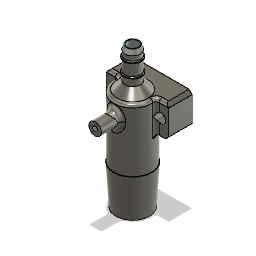
Pneumatic Connectors V2 - Respiratory Pressure V2 (Autodesk Fusion 360 design; units mm, degrees)
Autodesk Fusion 360 part; units mm, degrees
sketch "Sketch1" plane through (0, 0, 0) normal (0, 1, 0) x (1, 0, 0)
  circle A0 centre (0, 0) radius 5
  dimension "d1" = 10
  constraint coincident A0.centre origin
  measures "d1" diameter of A0
  measures "d21" distance of A0.centre
  measures "d24" diameter of A0.centre
  measures "d28" diameter of A0.centre
ref_plane "WorkPlane1" through (0, 15, 0) normal (0, 1, 0) x (1, 0, 0)
sketch "Sketch2" plane through (0, 15, 0) normal (0, 1, 0) x (1, 0, 0)
  circle A0 centre (0, 0) radius 5
  dimension "d3" = 10
  constraint coincident A0.centre origin
  measures "d3" diameter of A0
loft "Loft1" add profiles "Sketch1", "Sketch2" section 1 section 2
sketch "Sketch3" plane through (0, 15, 0) normal (0, 1, 0) x (-1, 0, 0)
  circle A0 centre (0, 0) radius 5
  circle A1 centre (0, 0) radius 3.5
  dimension "d4" = 7
  constraint coincident A0.centre A1.centre
  measures "d4" diameter of A1
sketch "Sketch4" plane through (0, 0, 0) normal (0, -1, 0) x (1, 0, 0)
  circle A0 centre (0, 0) radius 5
  circle A1 centre (0, 0) radius 3.5
  dimension "d5" = 7
  constraint concentric A0 A1
  measures "d5" diameter of A1
loft "Loft2" cut profiles "Sketch3", "Sketch4" section 1 contours A1 section 2 contours A1
sketch "Sketch14" plane through (0, 0, 0) normal (0, -1, 0) x (1, 0, 0)
  circle A0 centre (0, 0) radius 3.5
  circle A1 centre (0, 0) radius 5
  circle A2 centre (0, 0) radius 5
  constraint concentric A0 A2
  constraint equal A1 A2
extrude "Extrude2" add sketch "Sketch14" along normal blind 50
ref_plane "WorkPlane3" through (0, -75, 0) normal (0, -1, 0) x (1, 0, 0)
sketch "Sketch6" plane through (0, -75, 0) normal (0, -1, 0) x (1, 0, 0)
  circle A0 centre (0, 0) radius 10.75
  dimension "d42" = 21.5
  constraint coincident A0.centre origin
  measures "d42" diameter of A0
sketch "Sketch7" plane through (0, -50, 0) normal (0, -1, 0) x (1, 0, 0)
  circle A0 centre (0, 0) radius 3.5
  circle A1 centre (0, 0) radius 5
  circle A2 centre (0, 0) radius 12.25
  dimension "d43" = 24.5
  constraint concentric A0 A2
  measures "d43" diameter of A2
ref_plane "WorkPlane6" through (0, -50, 0) normal (0, -1, 0) x (1, 0, 0)
loft "Loft3" add profiles "Sketch7", "Sketch6" section 1 contours A1 | A2 section 2
sketch "Sketch8" plane through (0, -50, 0) normal (0, -1, 0) x (1, 0, 0)
  circle A0 centre (0, 0) radius 4.5
  dimension "d18" = 9
  constraint coincident A0.centre origin
  measures "d18" diameter of A0
sketch "Sketch15" plane through (0, -75, 0) normal (0, -1, 0) x (1, 0, 0)
  circle A0 centre (0, 0) radius 5.75
  circle A1 centre (0, 0) radius 11.75
  circle A2 centre (0, 0) radius 11.5
  circle A3 centre (0, 0) radius 7
  circle A4 centre (0, 0) radius 10.75
  dimension "d37" = 11.5
  measures "d37" diameter of A0
loft "Loft4" cut profiles "Sketch8", "Sketch15" section 1 section 2 contours A0
ref_plane "WorkPlane8" through (0, -10, 0) normal (0, -1, 0) x (1, 0, 0)
sketch "Sketch10" plane through (0, -10, 0) normal (0, -1, 0) x (1, 0, 0)
  line L0 (0, 0) -> (0, -30.326) construction
  line L1 (20, -3) -> (-20, -3)
  line L2 (-20, -3) -> (-20, -18)
  line L3 (-20, -18) -> (20, -18)
  line L4 (20, -18) -> (20, -3)
  line L5 (20, -3) -> (-20, -18) construction
  line L6 (-20, -3) -> (20, -18) construction
  circle A0 centre (0, 0) radius 5
  circle A1 centre (0, 0) radius 5
  point P0 (0, -10.5)
  dimension "d20" = 15
  dimension "d21" = 40
  constraint coincident L0.start A0.centre
  constraint vertical L0
  constraint horizontal L1
  constraint perpendicular L1 L2
  constraint parallel L1 L3
  constraint parallel L2 L4
  constraint coincident L5 P0
  constraint coincident L6 P0
  constraint coincident L0 P0
  measures "d20" distance of L1.start L3.end
  measures "d21" distance of L2.end L3.end
extrude "Extrude3" add sketch "Sketch10" along normal blind 20 contours L1 L2 L3 L4 A0 A1
sketch "Sketch11" plane through (0, 0, -3) normal (0, 0, 1) x (1, 0, 0)
  line L0 (-4, -10) -> (-20, -10)
  line L1 (-20, -30) -> (-4, -30)
  line L2 (-20, -10) -> (-20, -30)
  line L3 (-20, -20) -> (20, -20) construction
  line L4 (20, -30) -> (20, -10)
  circle A0 centre (0, -20) radius 15 construction
  circle A1 centre (-15, -20) radius 2.25
  circle A2 centre (15, -20) radius 2.25
  line L5 (-4, -30) -> (-4, -10)
  dimension "d24" = 4.5
  dimension "d25" = 5
  constraint midpoint L2 L3.start
  constraint perpendicular L2 L3
  constraint coincident L3.end L4
  constraint midpoint L3 A0.centre
  constraint coincident A0 A1.centre
  constraint coincident L3 A1.centre
  constraint coincident A0 A2.centre
  constraint coincident L3 A2.centre
  constraint equal A1 A2
  measures "d24" diameter of A2
  measures "d25" distance of L2 A1.centre
extrude "Extrude4" cut sketch "Sketch11" against normal up to surface (15 mm away) contours A1 | A2
sketch "Sketch12" plane through (0, 0, -3) normal (0, 0, 1) x (1, 0, 0)
  circle A0 centre (-15, -20) radius 2.25
  line L0 (-4, -10) -> (-20, -10)
  line L1 (-20, -30) -> (-4, -30)
  line L2 (-20, -10) -> (-20, -30)
  circle A1 centre (-15, -20) radius 3
  circle A2 centre (15, -20) radius 3
  circle A3 centre (15, -20) radius 2.25
  line L3 (-4, -30) -> (-4, -10)
  dimension "d28" = 6
  constraint concentric A0 A1
  constraint concentric A2 A3
  constraint equal A1 A2
  measures "d28" diameter of A2
extrude "Extrude5" cut sketch "Sketch12" against normal blind 9 contours A1 | A2
sketch "Sketch19" plane through (0, -50, 0) normal (0, 1, 0) x (-1, 0, 0)
  circle A0 centre (0, 0) radius 12.25
  circle A1 centre (0, 0) radius 12
  circle A2 centre (0, 0) radius 5
  dimension "d58" = 24
  constraint concentric A0 A1
  measures "d58" diameter of A1
extrude "Extrude10" add sketch "Sketch19" along normal up to surface (40 mm away) contours A1
sketch "Sketch20" plane through (0, 15, 0) normal (0, 1, 0) x (-1, 0, 0)
  circle A0 centre (0, 0) radius 3.5
  circle A1 centre (0, 0) radius 5
ref_plane "WorkPlane11" through (0, 8, 0) normal (0, 1, 0) x (-1, 0, 0)
sketch "Sketch21" plane through (0, 8, 0) normal (0, 1, 0) x (1, 0, 0)
  circle A0 centre (0, 0) radius 5
  circle A1 centre (0, 0) radius 5.5
  dimension "d62" = 11
  constraint concentric A0 A1
  measures "d62" diameter of A1
extrude "Extrude11" add sketch "Sketch21" along normal blind 1
ref_plane "WorkPlane12" through (0, -0.5, 0) normal (0, 1, 0) x (1, 0, 0)
sketch "Sketch22" plane through (0, -0.5, 0) normal (0, 1, 0) x (1, 0, 0)
  circle A0 centre (0, 0) radius 5.5
  circle A1 centre (0, 0) radius 5
extrude "Extrude12" add sketch "Sketch22" along normal blind 1
chamfer "Chamfer4" distance 0.5 angle 45 2 edges at (-5.1278, 0.5, 1.9889) (-5.1278, 9, 1.9889)
chamfer "Chamfer5" distance 3 distance2 1 1 edges at (-4.6616, 15, -1.8081) measured on face at (4.9938, 11, 0.2492)
chamfer "Chamfer6" distance 2 angle 45 4 edges at (20, -30, -10.5) (20, -10, -10.5) (-20, -30, -10.5) (-20, -10, -10.5)
fillet "Fillet2" radius 2 3 edges at (0, -30, -12) (11.619, -20, -3) (-11.619, -20, -3)
fillet "Fillet3" radius 2 5 edges at (15.9821, -10, -3) (12.5004, -10, -2.3628) (0, -10, 12) (-12.5004, -10, -2.3628) (-15.9821, -10, -3)
ref_plane "WorkPlane13" through (0, 0, 7) normal (0, 0, 1) x (1, 0, 0)
sketch "Sketch23" plane through (0, 0, 7) normal (0, 0, 1) x (1, 0, 0)
  circle A0 centre (-15, -20) radius 2.25
  line L0 (-15, -20) -> (15, -20) construction
  circle A1 centre (15, -20) radius 2.25
  circle A2 centre (0, -20) radius 4
  dimension "d74" = 8
  constraint coincident A0.centre L0.start
  constraint horizontal L0
  constraint coincident L0.end A1.centre
  constraint midpoint L0 A2.centre
  measures "d74" diameter of A2
extrude "Extrude13" add sketch "Sketch23" along normal blind 17 contours A2
sketch "Sketch24" plane through (0, 0, 24) normal (0, 0, 1) x (1, 0, 0)
  circle A0 centre (0, -20) radius 4
  circle A1 centre (0, -20) radius 1.5
  dimension "d78" = 3
  constraint concentric A0 A1
  measures "d78" diameter of A1
extrude "Extrude14" cut sketch "Sketch24" against normal blind 25 contours A1
ref_plane "WorkPlane14" through (0, -20, 22) normal (0, 0, 1) x (1, 0, 0)
sketch "Sketch25" plane through (0, -20, 22) normal (0, 0, 1) x (1, 0, 0)
  circle A0 centre (0, 0) radius 3
  circle A1 centre (0, 0) radius 4
  dimension "d82" = 6
  constraint coincident A0.centre A1.centre
  measures "d82" diameter of A0
extrude "Extrude15" add sketch "Sketch25" against normal blind 2 contours A0
chamfer "Chamfer7" [no effect]
fillet "Fillet4" radius 4 1 edges at (-4, -20, 11.3137)
chamfer "Chamfer8" distance 1 distance2 1 1 edges at (-4.1955, -50, -1.6273) measured on face at (4.1369, -50, -0.3974)
chamfer "Chamfer9" distance 5 angle 45 1 edges at (-4.6616, -10, 1.8081)
equation "d14 = 20 mm + 30 mm"
equation "d20 = 10 mm + 5 mm"
equation "d29 = -4 mm - 5 mm"
equation "d39 = -10 mm - 30 mm"
